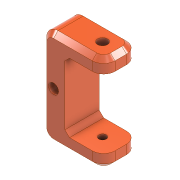
# Autodesk Inventor part: Print_Parts_I
Saved by Autodesk Inventor 2020.1 (Build 241239000, 239)
## iProperties
Created: 2020-09-30
Part Number: Print_Parts_I
Material: PC/ABS プラスチック
Document SubType Name: Modeling
Designer: kenta iguchi
Density: 0.357273 g/cm^3
Appearance: 滑らか - 淡いオレンジ
Author: kenta iguchi
Autodesk Inventor part; units mm, degrees
ref_plane "YZ Plane" through (0, 0, 0) normal (1, 0, 0) x (0, 1, 0)
ref_plane "XZ Plane" through (0, 0, 0) normal (0, 1, 0) x (-1, 0, 0)
ref_plane "XY Plane" through (0, 0, 0) normal (0, 0, 1) x (1, 0, 0)
sketch "スケッチ1" plane through (0, 0, 0) normal (0, 0, 1) x (1, 0, 0)
  line L0 (0, 21.1) -> (10, 21.1)
  line L1 (10, 21.1) -> (10, -21.1)
  line L2 (10, -21.1) -> (0, -21.1)
  line L3 (0, -21.1) -> (0, 21.1)
  line L4 (10, 21.1) -> (27, 21.1)
  line L5 (27, 21.1) -> (27, 15.1)
  line L6 (27, 15.1) -> (10, 15.1)
  line L7 (10, 15.1) -> (10, 21.1)
  line L8 (10, -21.1) -> (27, -21.1)
  line L9 (27, -21.1) -> (27, -15.1)
  line L10 (27, -15.1) -> (10, -15.1)
  line L11 (10, -15.1) -> (10, -21.1)
  point P0 (0, 0)
  point P1 (19, 15.1)
  point P2 (10, 15.1)
  dimension "d3" = 8
  dimension "d4" = 10
  dimension "d5" = 30.2
  dimension "d7" = 9
  dimension "d22" = 15.1
  dimension "d25" = 6
  dimension "d26" = 6
  constraints: 24 end point, 6 parallel, 3 horizontal, 3 perpendicular, 2 vertical alignment, 1 point on line
  measures "d3" distance from line of point (19, 15.1) L5
  measures "d4" distance between parallel lines of L3 L1
  measures "d5" distance between parallel lines of L6 L10
  measures "d7" distance from line of point (19, 15.1) L1
  measures "d22" distance from line of point (0, 0) L6
  measures "d25" distance of L4.end L5.end
  measures "d26" distance of L8.end L9.end
extrude "押し出し1" add sketch "スケッチ1" along normal blind 15
sketch "スケッチ2" plane through (0, 21.1, 0) normal (0, 1, 0) x (1, 0, 0)
  line L0 (27, -15) -> (0, -15) projected
  line L1 (27, 0) -> (27, -15) projected
  line L2 (27, 0) -> (10, 0) projected
  line L3 (10, 0) -> (10, -15) projected
  line L4 (27, -15) -> (10, -15) projected
  line L5 (27, 0) -> (27, -15) projected
  point P0 (19, -7.5)
  dimension "d10" = 8
  dimension "d11" = 7.5
  measures "d10" distance from line of point (19, -7.5) L1
  measures "d11" distance from line of L0 point (19, -7.5)
hole "穴1" at (19, 21.1, 7.5) direction (0, -1, 0) diameter 3.3 depth 58
sketch "スケッチ3" plane through (0, 21.1, 0) normal (0, 1, 0) x (1, 0, 0)
  circle A0 centre (19, -7.5) radius 1.65 projected
  circle A1 centre (19, -7.5) radius 2.2
  dimension "d19" = 4.4
  constraints: 1 centre point, 1 coincident
  measures "d19" diameter of A1
extrude "押し出し2" cut sketch "スケッチ3" against normal blind 10 contours A0 | A1
fillet "フィレット2" radius 5 6 edges at (27, 18.1, 0) (27, -18.1, 0) (27, -18.1, 15) (27, 18.1, 15) (0, 21.1, 7.5) (0, -21.1, 7.5)
sketch "スケッチ7" plane through (0, 0, 0) normal (0, 0, -1) x (-1, 0, 0)
  circle A0 centre (-5, 0) radius 2.2
  point P0 (0, 0)
  dimension "d55" = 4.4
  constraints: 1 centre point
  measures "d55" diameter of A0
extrude "押し出し5" cut sketch "スケッチ7" against normal blind 21.25
sketch "スケッチ8" plane through (0, 0, 0) normal (0, 0, -1) x (-1, 0, 0)
  circle A0 centre (-5, 0) radius 2.2 projected
  circle A1 centre (-5, 0) radius 1.75
  point P0 (0, 0)
  dimension "d65" = 3.5
  constraints: 1 centre point, 1 coincident
  measures "d65" diameter of A1
extrude "押し出し6" add sketch "スケッチ8" against normal blind 10
chamfer "面取り8" distance 0.45 angle 45 1 edges at (6.75, 0, 10)
chamfer "面取り9" distance 2 angle 45 16 edges at (13.5, 21.1, 15) (1.4645, 19.6355, 15) (0, 0, 15) (1.4645, -19.6355, 15) (13.5, -21.1, 15) (25.5355, -21.1, 13.5355) (27, -21.1, 7.5) (25.5355, -21.1, 1.4645) (13.5, -21.1, 0) (1.4645, -19.6355, 0) (0, 0, 0) (1.4645, 19.6355, 0) (13.5, 21.1, 0) (25.5355, 21.1, 1.4645) (27, 21.1, 7.5) (25.5355, 21.1, 13.5355)
chamfer "面取り10" distance 2 angle 45 2 edges at (10, -15.1, 7.5) (10, 15.1, 7.5)
sketch "スケッチ9" plane through (5, -21.1, 2) normal (0, -1, 0) x (1, 0, 0)
  circle A0 centre (14, 5.5) radius 1.65 projected
  point P0 (-5, -2)
hole "穴3" at (19, -21.1, 7.5) direction (0, 1, 0) diameter 6.5 depth 2
chamfer "面取り11" distance 0.5 angle 45 1 edges at (19, -21.1, 10.75)
equation "\"d22\" = 0.5 * d5"
